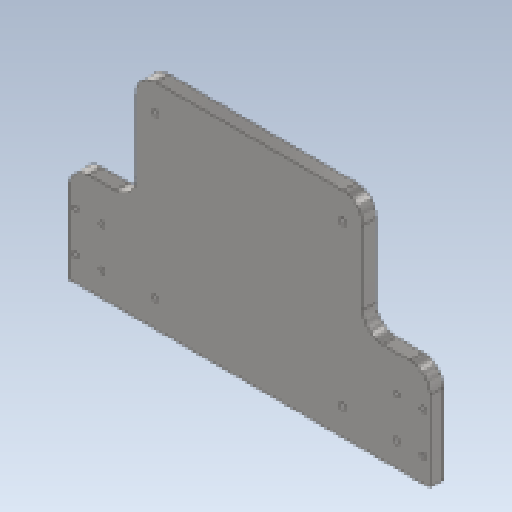
# Autodesk Inventor part: Support_lift
Saved by Autodesk Inventor 2025.2 (Build 292293000, 293)
## iProperties
Created: 2025-05-01
Part Number: Support_lift
Material: Stainless Steel
Document SubType Name: Modeling
Designer: Sergio Quintero
Density: 8 g/cm^3
Appearance: Semi-Polished
Author: Sergio Quintero
Autodesk Inventor part; units mm, degrees
ref_plane "YZ Plane" through (0, 0, 0) normal (1, 0, 0) x (0, 1, 0)
ref_plane "XZ Plane" through (0, 0, 0) normal (0, 1, 0) x (-1, 0, 0)
ref_plane "XY Plane" through (0, 0, 0) normal (0, 0, 1) x (1, 0, 0)
sketch "Sketch1" plane through (0, 0, 0) normal (0, 0, 1) x (1, 0, 0)
  line L0 (135, -80) -> (-135, -80)
  line L1 (-135, -80) -> (-135, 80)
  line L2 (-135, 80) -> (135, 80)
  line L3 (135, 80) -> (135, -80)
  line L4 (135, -80) -> (-135, 80) construction
  line L5 (-135, -80) -> (135, 80) construction
  point P0 (0, 0)
  dimension "d0" = 270
  dimension "d1" = 160
  constraints: 12 end point, 2 midpoint, 2 parallel, 1 horizontal, 1 perpendicular
  measures "d0" distance of L1.end L2.end
  measures "d1" distance of L0.end L1.end
extrude "Extrusion1" add sketch "Sketch1" along normal blind 10
sketch "Sketch2" plane through (0, 0, 10) normal (0, 0, 1) x (1, 0, 0)
  line L0 (70, -60) -> (-70, -60) construction
  line L1 (-70, -60) -> (-70, 60) construction
  line L2 (-70, 60) -> (70, 60) construction
  line L3 (70, 60) -> (70, -60) construction
  line L4 (70, -60) -> (-70, 60) construction
  line L5 (-70, -60) -> (70, 60) construction
  point P0 (0, 0)
  dimension "d4" = 140
  dimension "d5" = 120
  constraints: 12 end point, 4 coincident, 2 midpoint, 2 parallel, 1 horizontal, 1 perpendicular
  measures "d4" distance of L1.end L2.end
  measures "d5" distance of L0.end L1.end
hole "Hole1" at (-70, 60, 10) at (70, 60, 10) at (-70, -60, 10) at (70, -60, 10) direction (0, 0, -1) diameter 4.917 depth 25 tip angle 118 thread size "M6x1" class "6H" standard "ISO Metric profile"
sketch "Sketch3" plane through (0, 0, 0) normal (0, 0, -1) x (-1, 0, 0)
  line L0 (135, 80) -> (135, -80) construction
  line L1 (135, -80) -> (105, -80) construction
  line L2 (105, -80) -> (105, -20) construction
  line L3 (105, -20) -> (135, -20) construction
  line L4 (135, -20) -> (135, -80) construction
  line L5 (135, 80) -> (85, 80)
  line L6 (85, 80) -> (85, -5)
  line L7 (85, -5) -> (135, -5)
  line L8 (135, -5) -> (135, 80)
  point P0 (0, 0)
  dimension "d15" = 30
  dimension "d16" = 60
  dimension "d17" = 50
  dimension "d21" = 85
  constraints: 16 end point, 4 parallel, 2 horizontal, 2 perpendicular
  measures "d15" distance of L2.end L3.end
  measures "d16" distance of L1.end L2.end
  measures "d17" distance of L7.end L6.end
  measures "d21" distance between parallel lines of L7 L5
extrude "Extrusion2" cut sketch "Sketch3" against normal blind 10
fillet "Fillet2" radius 15 3 edges at (-85, 80, 5) (-85, -5, 5) (-135, -5, 5)
mirror "Mirror1" about plane through (0, 0, 0) normal (1, 0, 0) of "Extrusion2"
mirror "Mirror2" about plane through (0, 0, 0) normal (1, 0, 0) of "Fillet2"
sketch "Sketch4" plane through (0, 0, 0) normal (0, 0, -1) x (-1, 0, 0)
  line L0 (-130, -32) -> (-110, -32) construction
  line L1 (-110, -32) -> (-110, -62) construction
  line L2 (-110, -62) -> (-130, -62) construction
  line L3 (-130, -62) -> (-130, -32) construction
  line L4 (135, -80) -> (-135, -80) construction
  line L5 (-135, -80) -> (-135, -20) construction
  point P0 (0, 0)
  point P1 (-120, -62)
  point P2 (-130, -47)
  dimension "d22" = 20
  dimension "d23" = 30
  dimension "d24" = 18
  dimension "d25" = 5
  constraints: 8 end point, 4 coincident, 2 midpoint, 2 parallel, 1 horizontal, 1 perpendicular
  measures "d22" distance of L1.end L2.end
  measures "d23" distance of L0.end L1.end
  measures "d24" distance from line of L4 point (-120, -62)
  measures "d25" distance from line of L5 point (-130, -47)
hole "Hole2" at (130, -32, 0) at (110, -32, 0) at (110, -62, 0) at (130, -62, 0) direction (0, 0, 1) diameter 4.134 end through all thread size "M5x0.8" class "6H" standard "ISO Metric profile"
sketch "Sketch5" plane through (-135, -80, 0) normal (0, -1, 0) x (1, 0, 0)
  line L0 (270, 0) -> (270, 10) projected
  line L1 (0, 0) -> (270, 0) projected
  point P0 (135, 0)
  point P1 (255, 5)
  point P2 (270, 5)
  dimension "d33" = 15
  dimension "d34" = 5
  constraints: 1 midpoint
  measures "d33" distance of point (270, 5) point (255, 5)
  measures "d34" distance from line of L1 point (255, 5)
hole "Hole3" at (120, -80, 5) direction (0, 1, 0) diameter 4.917 depth 15 tip angle 118 thread size "M6x1" class "6H" standard "ISO Metric profile"
mirror "Mirror3" about plane through (0, 0, 0) normal (1, 0, 0) of "Hole2", "Hole3"
body "Solid1"
